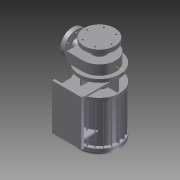
# Autodesk Inventor part: 液压泵
Saved by Autodesk Inventor 2012 (Build 160160000, 160)
## iProperties
Created: 2018-07-14
Part Number: 液压泵
Material: Default
Document SubType Name: Modeling
Designer: lxj
Density: 1 g/cm^3
Author: lxj
Autodesk Inventor part; units mm, degrees
ref_plane "YZ Plane" through (0, 0, 0) normal (1, 0, 0) x (0, 1, 0)
ref_plane "XZ Plane" through (0, 0, 0) normal (0, 1, 0) x (-1, 0, 0)
ref_plane "XY Plane" through (0, 0, 0) normal (0, 0, 1) x (1, 0, 0)
sketch "草图2" plane through (0, 0, 0) normal (0, 0, 1) x (1, 0, 0)
  circle A0 centre (0, 0) radius 125
  dimension "d0" = 250
  constraints: 1 centre point, 1 coincident
  measures "d0" diameter of A0
extrude "拉伸1" add sketch "草图2" against normal blind 20
sketch "草图3" plane through (0, 0, -20) normal (0, 0, -1) x (-1, 0, 0)
  circle A0 centre (0, 0) radius 125 projected
  circle A1 centre (0, 0) radius 105
  dimension "d3" = 210
  constraints: 1 centre point, 1 coincident
  measures "d3" diameter of A1
extrude "拉伸2" add sketch "草图3" along normal blind 250 contours A1
sketch "草图4" plane through (0, 0, -270) normal (0, 0, -1) x (-1, 0, 0)
  circle A0 centre (0, 0) radius 105 projected
  line L0 (0, 0) -> (241.1428, 0) construction
  line L1 (104.9952, -1) -> (123, -1)
  line L2 (123, -1) -> (123, 1)
  line L3 (123, 1) -> (104.9952, 1)
  point P0 (105, 0)
  dimension "d9" = 1
  dimension "d10" = 1
  dimension "d11" = 18
  constraints: 8 end point, 3 point on circle, 2 parallel, 1 horizontal, 1 perpendicular, 1 point on line
  measures "d9" distance between parallel lines of L3 L0
  measures "d10" distance between parallel lines of L1 L0
  measures "d11" distance from line of L2 point (105, 0)
extrude "拉伸3" add sketch "草图4" against normal blind 250 contours A0 L3 L2 L1
pattern_circular "环形阵列1" count 20 over 360 about axis through (0, 0, -20) along (0, 0, -1) of "拉伸3"
sketch "草图5" plane through (0, 0, -270) normal (0, 0, -1) x (-1, 0, 0)
  arc A0 (85.5307, -60.9056) -> (99.5474, -33.3964) centre (0, 0) ccw projected
  circle A1 centre (0, 0) radius 125
  dimension "d17" = 250
  constraints: 1 centre point, 1 coincident
  measures "d17" diameter of A1
extrude "拉伸4" add sketch "草图5" along normal blind 40
fillet "圆角1" radius 20 1 edges at (125, 0, -310)
sketch "草图6" plane through (0, 0, 0) normal (0, 0, 1) x (1, 0, 0)
  circle A0 centre (0, 0) radius 125 projected
  circle A1 centre (0, 0) radius 60
  dimension "d21" = 120
  constraints: 1 centre point, 1 coincident
  measures "d21" diameter of A1
extrude "拉伸5" add sketch "草图6" along normal blind 80 contours A1
sketch "草图7" plane through (0, 0, 0) normal (0, 0, 1) x (1, 0, 0)
  circle A0 centre (0, 0) radius 60 projected
  circle A1 centre (0, 0) radius 125 projected
  line L0 (90.252, 7.5987) -> (90.252, 7.5831)
  line L1 (59.5169, 7.5831) -> (59.5169, 7.5987)
  line L2 (59.7913, 5) -> (114.7913, 5)
  line L3 (114.7913, 5) -> (114.7913, -5)
  line L4 (114.7913, -5) -> (59.7913, -5)
  line L5 (0, 0) -> (125, 0) construction
  dimension "d24" = 55
  dimension "d25" = 5
  dimension "d26" = 5
  constraints: 12 end point, 3 perpendicular, 3 point on circle, 1 horizontal, 1 horizontal alignment, 1 parallel, 1 other
  measures "d24" distance of L3.end L4.end
  measures "d25" distance between parallel lines of L5 L2
  measures "d26" distance between parallel lines of L5 L4
extrude "拉伸6" add sketch "草图7" along normal blind 80 contours A0 L2 L3 L4
pattern_circular "环形阵列2" count 4 over 360 about axis through (0, 0, -20) along (0, 0, -1) of "拉伸6"
sketch "草图8" plane through (0, 0, 80) normal (0, 0, 1) x (1, 0, 0)
  arc A0 (-59.7913, -5) -> (-5, -59.7913) centre (0, 0) ccw projected
  circle A1 centre (0, 0) radius 125
  dimension "d32" = 250
  constraints: 1 centre point, 1 coincident
  measures "d32" diameter of A1
extrude "拉伸7" add sketch "草图8" along normal blind 20
sketch "草图9" plane through (0, 0, 100) normal (0, 0, 1) x (1, 0, 0)
  circle A0 centre (0, 0) radius 125 projected
  arc A1 (0, -100) -> (0, 100) centre (0, 0) ccw
  line L0 (0, 100) -> (-100, 100)
  line L1 (-100, 100) -> (-100, -100)
  line L2 (-100, -100) -> (0, -100)
  dimension "d35" = 100
  dimension "d36" = 100
  constraints: 6 end point, 2 point on circle, 2 tangent, 1 centre point, 1 coincident, 1 horizontal, 1 parallel, 1 perpendicular
  measures "d35" radius of A1
  measures "d36" distance of L0.start L0.end
extrude "拉伸8" add sketch "草图9" along normal blind 60 contours L0 A1 L2 A0 L1 | A0 L1 L0 | L2 L1 A0
sketch "草图10" plane through (0, 0, 160) normal (0, 0, 1) x (1, 0, 0)
  arc A0 (0, -100) -> (0, 100) centre (0, 0) ccw projected
  circle A1 centre (0, 0) radius 42.5
  dimension "d39" = 85
  constraints: 1 centre point, 1 coincident
  measures "d39" diameter of A1
extrude "拉伸9" add sketch "草图10" along normal blind 50
sketch "草图11" plane through (0, 0, 210) normal (0, 0, 1) x (1, 0, 0)
  circle A0 centre (0, 0) radius 42.5 projected
  circle A1 centre (0, 0) radius 95
  dimension "d42" = 190
  constraints: 1 centre point, 1 coincident
  measures "d42" diameter of A1
extrude "拉伸10" add sketch "草图11" along normal blind 25 contours A0 | A1
sketch "草图12" plane through (0, 0, 235) normal (0, 0, 1) x (1, 0, 0)
  circle A0 centre (0, 0) radius 95 projected
  circle A1 centre (75, 0) radius 5
  dimension "d26" = 5
  dimension "d45" = 75
  dimension "d46" = 10
  constraints: 1 centre point
  measures "d45" distance of A1.centre A0.centre
  measures "d46" diameter of A1
extrude "拉伸11" cut sketch "草图12" against normal blind 25 contours A1
pattern_circular "环形阵列3" count 6 over 360 about axis through (0, 0, -20) along (0, 0, -1) of "拉伸11"
sketch "草图13" plane through (-100, 75, 100) normal (-1, 0, 0) x (0, 0, 1)
  line L0 (0, -175) -> (60, -175) projected
  circle A0 centre (30, -75) radius 30
  point P0 (-100, -75)
  dimension "d52" = 100
  dimension "d53" = 60
  constraints: 1 centre point
  measures "d52" distance from line of L0 A0.centre
  measures "d53" diameter of A0
extrude "拉伸12" add sketch "草图13" along normal blind 40
sketch "草图14" plane through (-140, 0, 130) normal (-1, 0, 0) x (0, 0, 1)
  circle A0 centre (0, 0) radius 30 projected
  circle A1 centre (0, 0) radius 75
  point P0 (-130, 0)
  dimension "d56" = 150
  constraints: 1 centre point, 1 coincident
  measures "d56" diameter of A1
extrude "拉伸13" add sketch "草图14" along normal blind 25 contours A0 | A1
sketch "草图15" plane through (-165, 0, 130) normal (-1, 0, 0) x (0, 0, 1)
  circle A0 centre (0, 0) radius 75 projected
  circle A1 centre (60, 0) radius 5
  point P0 (-130, 0)
  dimension "d59" = 60
  dimension "d60" = 10
  constraints: 1 centre point
  measures "d59" distance of A1.centre A0.centre
  measures "d60" diameter of A1
extrude "拉伸14" cut sketch "草图15" against normal blind 25 contours A1
pattern_circular "环形阵列4" count 6 over 360 about axis through (-140, 0, 130) along (-1, 0, 0) of "拉伸14"
sketch "草图16" plane through (-114.7913, -5, 0) normal (0, -1, 0) x (1, 0, 0)
  line L0 (55, 80) -> (0, 80) projected
  line L1 (44.7913, 35) -> (184.7913, 35)
  line L2 (184.7913, 35) -> (184.7913, 25)
  line L3 (184.7913, 25) -> (44.7913, 25)
  line L4 (44.7913, 25) -> (44.7913, 35)
  line L5 (44.7913, -185) -> (184.7913, -185)
  line L6 (184.7913, -185) -> (184.7913, -195)
  line L7 (184.7913, -195) -> (44.7913, -195)
  line L8 (44.7913, -195) -> (44.7913, -185)
  point P0 (114.7913, 0)
  dimension "d66" = 45
  dimension "d67" = 265
  dimension "d68" = 140
  dimension "d69" = 10
  dimension "d70" = 70
  dimension "d71" = 140
  dimension "d72" = 10
  dimension "d73" = 70
  constraints: 16 end point, 4 parallel, 2 horizontal, 2 perpendicular
  measures "d66" distance between parallel lines of L1 L0
  measures "d67" distance between parallel lines of L5 L0
  measures "d68" distance of L2.end L3.end
  measures "d69" distance of L1.end L2.end
  measures "d70" distance from line of point (114.791, 0) L4
  measures "d71" distance of L6.end L7.end
  measures "d72" distance of L7.end L5.start
  measures "d73" distance from line of L8 point (114.791, 0)
extrude "拉伸15" add sketch "草图16" along normal blind 180
sketch "草图17" plane through (-114.7913, -185, 0) normal (0, -1, 0) x (1, 0, 0)
  line L0 (24.7913, 60) -> (204.7913, 60)
  line L1 (204.7913, 60) -> (204.7913, -220)
  line L2 (204.7913, -220) -> (24.7913, -220)
  line L3 (24.7913, -220) -> (24.7913, 60)
  line L4 (184.7913, -195) -> (44.7913, -195) projected
  point P0 (114.7913, 0)
  dimension "d76" = 280
  dimension "d77" = 180
  dimension "d78" = 90
  dimension "d79" = 25
  constraints: 8 end point, 2 parallel, 1 horizontal, 1 perpendicular
  measures "d76" distance of L0.end L1.end
  measures "d77" distance of L1.end L2.end
  measures "d78" distance from line of L1 point (114.791, 0)
  measures "d79" distance between parallel lines of L4 L2
extrude "Sur" add sketch "草图17" along normal blind 15
